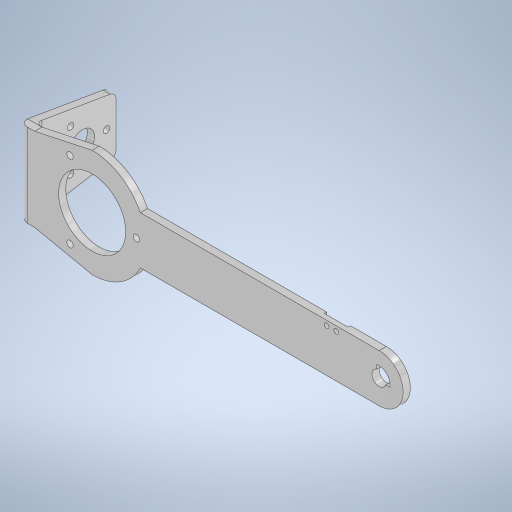
# Autodesk Inventor part: motor_holder_1
Saved by Autodesk Inventor 2024 (Build 280153000, 153)
## iProperties
Created: 2025-02-07
Part Number: motor_holder_1
Material: アルミニウム 6061
Document SubType Name: Modeling
Designer: 1412z
Density: 2.7 g/cm^3
Appearance: アルミニウム - つや出し
Author: 1412z
Autodesk Inventor part; units mm, degrees
ref_plane "YZ Plane" through (0, 0, 0) normal (1, 0, 0) x (0, 1, 0)
ref_plane "XZ Plane" through (0, 0, 0) normal (0, 1, 0) x (-1, 0, 0)
ref_plane "XY Plane" through (0, 0, 0) normal (0, 0, 1) x (1, 0, 0)
sketch "スケッチ1" plane through (0, 0, 0) normal (1, 0, 0) x (0, 1, 0)
  circle A0 centre (0, 0) radius 10
  circle A1 centre (0, -10) radius 1.35
  circle A2 centre (8.6603, 5) radius 1.35
  circle A3 centre (-8.6603, 5) radius 1.35
  circle A4 centre (0, 0) radius 5
  line L0 (0, 0) -> (0, 50)
  circle A5 centre (0, 50) radius 22.5
  circle A6 centre (0, 0) radius 14
  line L1 (-14, 0) -> (-22.5, 50)
  line L2 (14, 0) -> (22.5, 50)
  line L3 (0, -14) -> (-11.62, -14)
  line L4 (-11.62, -14) -> (-14, 0)
  line L5 (0, -14) -> (11.62, -14)
  line L6 (11.62, -14) -> (14, 0)
  line L7 (0, 20) -> (-17.4, 20)
  line L8 (0, 20) -> (17.4, 20)
  dimension "d0" = 20
  dimension "d1" = 2.7
  dimension "d4" = 360
  dimension "d6" = 10
  dimension "d7" = 50
  dimension "d8" = 45
  dimension "d9" = 28
  constraints: 18 end point, 7 point on line, 6 centre point, 6 coincident, 5 point on circle, 1 horizontal, 1 perpendicular, 1 tangent, 1 vertical, 1 vertical alignment, 10 other
  measures "d1" diameter of A1
  measures "d6" diameter of A4
  measures "d7" distance of L0.start L0.end
  measures "d8" diameter of A5
  measures "d9" diameter of A6
extrude "押し出し1" add sketch "スケッチ1" along normal blind 3 contours A0 A1 A3 A2 | A6 L6 L4 | A6 L1 L7 L0 | L0 L8 L2 A6 | L6 L5 A6 | A6 L3 L4
sketch "スケッチ2" plane through (0, -17.4, 20) normal (0, 0, 1) x (1, 0, 0)
  line L0 (0, 17.4) -> (30, 17.4)
  circle A0 centre (30, 17.4) radius 22.5
  circle A1 centre (30, 17.4) radius 18.5
  circle A2 centre (30, 17.4) radius 14
  circle A3 centre (48.5, 17.4) radius 1.35
  circle A4 centre (20.75, 33.4215) radius 1.35
  circle A5 centre (20.75, 1.3785) radius 1.35
  line L1 (0, 29.02) -> (0, 34.8) projected
  line L2 (0, 0) -> (0, 5.78) projected
  line L3 (0, 34.8) -> (0, 0)
  line L4 (3, 29.02) -> (3, 34.8) projected
  line L5 (3, 34.8) -> (6, 34.8)
  line L6 (6, 34.8) -> (30, 39.9)
  line L7 (3, 0) -> (3, 5.78) projected
  line L8 (3, 0) -> (6, 0)
  line L9 (6, 0) -> (30, -5.1)
  line L10 (3, 0) -> (0, 0)
  line L11 (0, 34.8) -> (3, 34.8) projected
  line L12 (0, 0) -> (0, 34.8)
  line L13 (0, 34.8) -> (3, 34.8)
  dimension "d14" = 37
  dimension "d12" = 30
  dimension "d13" = 45
  dimension "d15" = 28
  dimension "d16" = 2.7
  dimension "d19" = 360
  dimension "d21" = 3
  dimension "d22" = 3
  constraints: 18 end point, 5 centre point, 4 horizontal, 3 coincident, 2 point on circle, 1 collinear, 1 horizontal alignment, 1 perpendicular, 1 vertical, 9 other
  measures "d12" distance of L0.start L0.end
  measures "d13" diameter of A0
  measures "d15" diameter of A2
  measures "d16" diameter of A3
  measures "d21" distance of L4.end L5.end
  measures "d22" distance of L7.start L8.end
extrude "押し出し2" add sketch "スケッチ2" along normal blind 3 contours L3 L1 L11 L5 L6 A0 L0 | L0 A0 L9 L8 L10 L2 L3 | A1 A4 A3 A5 | A0 L6 L9
fillet "フィレット1" radius 3 2 edges at (3, 0, 20) (0, 0, 23)
fillet "フィレット2" radius 3 2 edges at (1.5, -11.62, -14) (1.5, 11.62, -14)
sketch "スケッチ3" plane through (0, -17.4, 23) normal (0, 0, 1) x (1, 0, 0)
  arc A0 (30, -5.1) -> (30, 39.9) centre (30, 17.4) ccw projected
  line L0 (30, 17.4) -> (150, 17.4)
  circle A1 centre (150, 17.4) radius 10
  line L1 (150, 27.4) -> (50.1556, 27.4)
  line L2 (150, 7.4) -> (50.1556, 7.4)
  circle A2 centre (150, 17.4) radius 3
  line L3 (150, 17.4) -> (150, 16.4)
  line L4 (150, 16.4) -> (154.5, 16.4)
  line L5 (150, 17.4) -> (149, 17.4)
  line L6 (149, 17.4) -> (149, 21.9)
  arc A3 (154.5, 16.4) -> (149, 21.9) centre (149.3141, 16.7141) ccw
  point P0 (0, 17.4)
  dimension "d27" = 120
  dimension "d28" = 20
  dimension "d29" = 6
  dimension "d32" = 1
  dimension "d33" = 4.5
  dimension "d34" = 1
  dimension "d35" = 4.5
  constraints: 14 end point, 6 point on circle, 3 centre point, 2 coincident, 2 parallel, 2 perpendicular, 1 horizontal, 1 point on line, 1 tangent, 1 vertical
  measures "d27" distance of L0.start L0.end
  measures "d28" diameter of A1
  measures "d29" diameter of A2
  measures "d32" distance of L3.start L3.end
  measures "d33" distance of L3.end L4.end
  measures "d34" distance of L3.start L5.end
  measures "d35" distance of L5.end L6.end
extrude "押し出し3" add sketch "スケッチ3" against normal blind 3 contours A0 L0 A1 L2 | A0 L1 A1 L0 | A1 | L6 A3 L4 A2
sketch "スケッチ4" plane through (0, -17.4, 23) normal (0, 0, 1) x (1, 0, 0)
  circle A0 centre (150, 17.4) radius 3 projected
  line L0 (150, 17.4) -> (150, 16.4)
  line L1 (150, 16.4) -> (154.5, 16.4)
  line L2 (150, 17.4) -> (154.5, 17.4)
  line L3 (150, 17.4) -> (149, 17.4)
  line L4 (149, 17.4) -> (149, 21.9)
  line L5 (150, 17.4) -> (150, 21.9)
  line L6 (149, 21.9) -> (150, 21.9)
  line L7 (154.5, 17.4) -> (154.5, 16.4)
  arc A1 (154.5, 17.4) -> (150, 21.9) centre (150, 17.4) ccw
  point P0 (0, 17.4)
  point P1 (149, 20.2284)
  point P2 (152.8284, 16.4)
  dimension "d36" = 1
  dimension "d37" = 4.5
  dimension "d38" = 1
  dimension "d39" = 4.5
  constraints: 16 end point, 3 horizontal, 3 perpendicular, 2 point on circle, 2 vertical, 1 centre point, 1 tangent
  measures "d36" distance of L0.start L0.end
  measures "d37" distance of L0.end L1.end
  measures "d38" distance of L0.start L3.end
  measures "d39" distance of L3.end L4.end
extrude "押し出し4" cut sketch "スケッチ4" against normal blind 3 contours L2 L7 L1 A0 | A0 L5 A1 L2 | A0 L4 L6 L5
sketch "スケッチ5" plane through (0, -17.4, 23) normal (0, 0, 1) x (1, 0, 0)
  circle A0 centre (132, 25.4) radius 1
  circle A1 centre (128, 25.4) radius 1
  point P0 (0, 17.4)
  dimension "d42" = 2
  dimension "d43" = 2
  constraints: 2 centre point
  measures "d42" diameter of A0
  measures "d43" diameter of A1
extrude "押し出し5" cut sketch "スケッチ5" against normal blind 3
thread "ねじ1" size "M2x0.4" class "6H" standard "ANSI Metric M Profile" full length
thread "ねじ2" size "M2x0.4" class "6H" standard "ANSI Metric M Profile" full length
sketch "スケッチ6" plane through (0, -17.4, 20) normal (0, 0, -1) x (-1, 0, 0)
  line L0 (-50.1556, 27.4) -> (-150, 27.4) projected
  line L1 (-130, 27.4) -> (-125, 27.4)
  line L2 (-125, 27.4) -> (-125, 22.4)
  line L3 (-125, 22.4) -> (-135, 22.4)
  line L4 (-135, 22.4) -> (-135, 27.4)
  line L5 (-135, 27.4) -> (-130, 27.4)
  point P0 (0, 17.4)
  dimension "d50" = 5
  dimension "d51" = 5
  dimension "d52" = 10
  constraints: 10 end point, 4 perpendicular, 3 point on line
  measures "d50" distance of L1.start L1.end
  measures "d51" distance of L1.end L2.end
  measures "d52" distance of L2.end L3.end
extrude "押し出し6" cut sketch "スケッチ6" against normal blind 1
